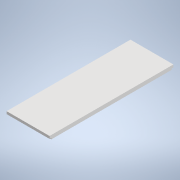
# Autodesk Inventor part: Arcade_MonitorMount
Saved by Autodesk Inventor 2022 (Build 260153000, 153)
## iProperties
Created: 2023-12-22
Part Number: Arcade_MonitorMount
Material: Generic
Document SubType Name: Modeling
Designer: Petr Černý
Density: 1 g/cm^3
Appearance: Default
Author: Petr Černý
Autodesk Inventor part; units mm, degrees
ref_plane "YZ Plane" through (0, 0, 0) normal (1, 0, 0) x (0, 1, 0)
ref_plane "XZ Plane" through (0, 0, 0) normal (0, 1, 0) x (-1, 0, 0)
ref_plane "XY Plane" through (0, 0, 0) normal (0, 0, 1) x (1, 0, 0)
sketch "Sketch1" plane through (0, 0, 0) normal (0, 1, 0) x (-1, 0, 0)
  line L0 (18.603, 38.914) -> (-151.397, 38.914)
  line L1 (-151.397, 38.914) -> (-151.397, -451.086)
  line L2 (-151.397, -451.086) -> (18.603, -451.086)
  line L3 (18.603, -451.086) -> (18.603, 38.914)
  point P0 (0, 0)
  dimension "d0" = 170
  dimension "d1" = 490
  constraints: 8 end point, 2 parallel, 1 horizontal, 1 perpendicular
  measures "d0" distance of L2.end L1.end
  measures "d1" distance of L1.end L0.end
extrude "Extrusion1" add sketch "Sketch1" along normal blind 15
sketch "Sketch2" plane through (-18.603, 0, 38.914) normal (0, 0, 1) x (1, 0, 0)
  line L0 (170, 0) -> (0, 0) projected
  line L1 (0, 0) -> (170, 0)
  line L2 (170, 0) -> (170, 5)
  line L3 (170, 5) -> (0, 5)
  line L4 (0, 5) -> (0, 0)
  point P0 (18.603, 0)
  dimension "d4" = 170
  dimension "d5" = 5
  constraints: 8 end point, 2 parallel, 1 horizontal, 1 perpendicular
  measures "d4" distance of L3.end L2.end
  measures "d5" distance of L2.end L1.end
extrude "Extrusion2" cut sketch "Sketch2" against normal blind 7
sketch "Sketch3" plane through (151.397, 0, -451.086) normal (0, 0, -1) x (-1, 0, 0)
  line L0 (0, 0) -> (170, 0) projected
  line L1 (0, 0) -> (170, 0)
  line L2 (170, 0) -> (170, 5)
  line L3 (170, 5) -> (0, 5)
  line L4 (0, 5) -> (0, 0)
  point P0 (151.397, 0)
  dimension "d8" = 170
  dimension "d9" = 5
  constraints: 8 end point, 2 parallel, 1 horizontal, 1 perpendicular
  measures "d8" distance of L3.end L2.end
  measures "d9" distance of L2.end L1.end
extrude "Extrusion3" cut sketch "Sketch3" against normal blind 7
body "Solid1"
